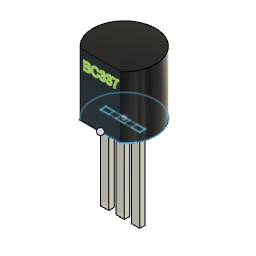
BC337 (Autodesk Fusion 360 design; units mm, degrees)
Autodesk Fusion 360 part; units mm, degrees
sketch "Sketch1" plane through (0, 0, 0) normal (0, 0, 1) x (1, 0, 0)
  line L0 (0, 0) -> (-1.725, 0)
  line L1 (-1.725, 0) -> (-1.725, 0.0215)
  line L2 (1.725, 0) -> (1.725, 0.0215)
  line L3 (0, 0) -> (1.725, 0)
  arc A0 (1.7, 0) -> (-1.7, 0) centre (0, 2) ccw
  line L4 (-1.6, 1.6) -> (1.7, 1.6)
  line L5 (1.7, 1.6) -> (1.7, 2.05)
  line L6 (1.7, 2.05) -> (-1.6, 2.05)
  line L7 (-1.6, 2.05) -> (-1.6, 1.6)
  line L8 (-1.6, 1.6) -> (-0.9, 1.6)
  line L9 (-0.9, 1.6) -> (-0.9, 2.05)
  line L10 (-0.9, 2.05) -> (-1.6, 2.05)
  line L11 (-1.6, 2.05) -> (-1.6, 1.6)
  line L12 (1.7, 2.05) -> (1, 2.05)
  line L13 (1, 2.05) -> (1, 1.6)
  line L14 (1, 1.6) -> (1.7, 1.6)
  line L15 (1.7, 1.6) -> (1.7, 2.05)
  line L16 (-0.2974, 2.05) -> (0.4026, 2.05)
  line L17 (0.4026, 2.05) -> (0.4026, 1.6)
  line L18 (0.4026, 1.6) -> (-0.2974, 1.6)
  line L19 (-0.2974, 1.6) -> (-0.2974, 2.05)
  dimension "d7" = 3.3
  dimension "d8" = 0.45
  dimension "d9" = 0.7
  dimension "d10" = 0.7
  dimension "d11" = 0.7
  constraint coincident L0.start L3.start
  constraint horizontal L0
  constraint perpendicular L0 L1
  constraint coincident L0 A0.end
  constraint coincident L3 A0.start
  constraint coincident A0 L1.end
  constraint coincident A0 L2.end
  constraint horizontal L4
  constraint vertical L5
  constraint horizontal L6
  constraint vertical L7
  constraint horizontal L8
  constraint vertical L9
  constraint horizontal L10
  constraint vertical L11
  constraint horizontal L12
  constraint vertical L13
  constraint horizontal L14
  constraint vertical L15
  constraint horizontal L16
  constraint vertical L17
  constraint horizontal L18
  constraint vertical L19
  constraint coincident L6 L16.start
  measures "d7" distance of L4.start L4.end
  measures "d8" distance of L4.start L6.end
  measures "d9" distance of L4.start L8.end
  measures "d10" distance of L5.end L12.end
  measures "d11" distance of L16.start L16.end
extrude "Extrude2" add sketch "Sketch1" against normal blind 7 contours L4 L5 L6 L12 L13 L14 L15 makes body 1
extrude "Extrude1" add sketch "Sketch1" along normal blind 5.2 separate body contours L0 L3 A0 | L4 L6 L7 L8 L9 L10 L11 | L4 L6 L9 L19 | L4 L6 L16 L17 L18 L19 | L4 L6 L13 L17 | L4 L5 L6 L12 L13 L14 L15 makes body 2
extrude "Extrude3" add sketch "Sketch1" against normal blind 7 contours L4 L6 L16 L17 L18 L19 bodies 2
extrude "Extrude4" add sketch "Sketch1" against normal blind 7 contours L4 L6 L7 L8 L9 L10 L11 bodies 2
sketch "Sketch2" plane through (0, 0, 0) normal (0, -1, 0) x (1, 0, 0)
  line L0 (-1.7, 0) -> (1.7, 0)
  line L1 (1.7, 0) -> (1.7, 5.2)
  line L2 (1.7, 5.2) -> (-1.7, 5.2)
  line L3 (-1.7, 5.2) -> (-1.7, 0)
  line L4 (-1.3801, 3.7908) -> (-1.3801, 4.4908)
  line L5 (-1.3801, 4.4908) -> (-1.1175, 4.4908)
  spline S0 degree 2 poles (-1.1175, 4.4908) (-1.0373, 4.4908) (-0.9888, 4.4696) knots 0 0 0 1 1 1
  spline S1 degree 2 poles (-0.9888, 4.4696) (-0.9403, 4.4483) (-0.9129, 4.4042) knots 0 0 0 1 1 1
  spline S2 degree 2 poles (-0.9129, 4.4042) (-0.8854, 4.36) (-0.8854, 4.3118) knots 0 0 0 1 1 1
  spline S3 degree 2 poles (-0.8854, 4.3118) (-0.8854, 4.2669) (-0.9098, 4.2273) knots 0 0 0 1 1 1
  spline S4 degree 2 poles (-0.9098, 4.2273) (-0.9341, 4.1876) (-0.9833, 4.1633) knots 0 0 0 1 1 1
  spline S5 degree 2 poles (-0.9833, 4.1633) (-0.9198, 4.1447) (-0.8857, 4.0998) knots 0 0 0 1 1 1
  spline S6 degree 2 poles (-0.8857, 4.0998) (-0.8515, 4.0549) (-0.8515, 3.9938) knots 0 0 0 1 1 1
  spline S7 degree 2 poles (-0.8515, 3.9938) (-0.8515, 3.9446) (-0.8723, 3.9023) knots 0 0 0 1 1 1
  spline S8 degree 2 poles (-0.8723, 3.9023) (-0.8931, 3.8601) (-0.9236, 3.8372) knots 0 0 0 1 1 1
  spline S9 degree 2 poles (-0.9236, 3.8372) (-0.9542, 3.8142) (-1.0003, 3.8025) knots 0 0 0 1 1 1
  spline S10 degree 2 poles (-1.0003, 3.8025) (-1.0463, 3.7908) (-1.1132, 3.7908) knots 0 0 0 1 1 1
  line L6 (-1.1132, 3.7908) -> (-1.3801, 3.7908)
  line L7 (-1.2875, 4.1967) -> (-1.1361, 4.1967)
  spline S11 degree 2 poles (-1.1361, 4.1967) (-1.0745, 4.1967) (-1.0478, 4.2048) knots 0 0 0 1 1 1
  spline S12 degree 2 poles (-1.0478, 4.2048) (-1.0124, 4.2153) (-0.9945, 4.2397) knots 0 0 0 1 1 1
  spline S13 degree 2 poles (-0.9945, 4.2397) (-0.9766, 4.264) (-0.9766, 4.3008) knots 0 0 0 1 1 1
  spline S14 degree 2 poles (-0.9766, 4.3008) (-0.9766, 4.3357) (-0.9933, 4.3622) knots 0 0 0 1 1 1
  spline S15 degree 2 poles (-0.9933, 4.3622) (-1.01, 4.3887) (-1.0411, 4.3984) knots 0 0 0 1 1 1
  spline S16 degree 2 poles (-1.0411, 4.3984) (-1.0721, 4.4082) (-1.1476, 4.4082) knots 0 0 0 1 1 1
  line L8 (-1.1476, 4.4082) -> (-1.2875, 4.4082)
  line L9 (-1.2875, 4.4082) -> (-1.2875, 4.1967)
  line L10 (-1.2875, 3.8734) -> (-1.1132, 3.8734)
  spline S17 degree 2 poles (-1.1132, 3.8734) (-1.0683, 3.8734) (-1.0502, 3.8768) knots 0 0 0 1 1 1
  spline S18 degree 2 poles (-1.0502, 3.8768) (-1.0182, 3.8825) (-0.9967, 3.8959) knots 0 0 0 1 1 1
  spline S19 degree 2 poles (-0.9967, 3.8959) (-0.9752, 3.9093) (-0.9613, 3.9348) knots 0 0 0 1 1 1
  spline S20 degree 2 poles (-0.9613, 3.9348) (-0.9475, 3.9603) (-0.9475, 3.9938) knots 0 0 0 1 1 1
  spline S21 degree 2 poles (-0.9475, 3.9938) (-0.9475, 4.0329) (-0.9676, 4.0618) knots 0 0 0 1 1 1
  spline S22 degree 2 poles (-0.9676, 4.0618) (-0.9876, 4.0907) (-1.0232, 4.1024) knots 0 0 0 1 1 1
  spline S23 degree 2 poles (-1.0232, 4.1024) (-1.0588, 4.1141) (-1.1256, 4.1141) knots 0 0 0 1 1 1
  line L11 (-1.1256, 4.1141) -> (-1.2875, 4.1141)
  line L12 (-1.2875, 4.1141) -> (-1.2875, 3.8734)
  line L13 (-0.2246, 4.0363) -> (-0.1319, 4.0129)
  spline S24 degree 2 poles (-0.1319, 4.0129) (-0.1611, 3.8988) (-0.2368, 3.8388) knots 0 0 0 1 1 1
  spline S25 degree 2 poles (-0.2368, 3.8388) (-0.3124, 3.7789) (-0.4218, 3.7789) knots 0 0 0 1 1 1
  spline S26 degree 2 poles (-0.4218, 3.7789) (-0.5349, 3.7789) (-0.6059, 3.825) knots 0 0 0 1 1 1
  spline S27 degree 2 poles (-0.6059, 3.825) (-0.6768, 3.8711) (-0.7138, 3.9584) knots 0 0 0 1 1 1
  spline S28 degree 2 poles (-0.7138, 3.9584) (-0.7508, 4.0458) (-0.7508, 4.1461) knots 0 0 0 1 1 1
  spline S29 degree 2 poles (-0.7508, 4.1461) (-0.7508, 4.2554) (-0.709, 4.3368) knots 0 0 0 1 1 1
  spline S30 degree 2 poles (-0.709, 4.3368) (-0.6672, 4.4183) (-0.5901, 4.4605) knots 0 0 0 1 1 1
  spline S31 degree 2 poles (-0.5901, 4.4605) (-0.513, 4.5028) (-0.4203, 4.5028) knots 0 0 0 1 1 1
  spline S32 degree 2 poles (-0.4203, 4.5028) (-0.3153, 4.5028) (-0.2437, 4.4493) knots 0 0 0 1 1 1
  spline S33 degree 2 poles (-0.2437, 4.4493) (-0.1721, 4.3958) (-0.1439, 4.2989) knots 0 0 0 1 1 1
  line L14 (-0.1439, 4.2989) -> (-0.2351, 4.2774)
  spline S34 degree 2 poles (-0.2351, 4.2774) (-0.2594, 4.3538) (-0.3058, 4.3887) knots 0 0 0 1 1 1
  spline S35 degree 2 poles (-0.3058, 4.3887) (-0.3521, 4.4235) (-0.4223, 4.4235) knots 0 0 0 1 1 1
  spline S36 degree 2 poles (-0.4223, 4.4235) (-0.503, 4.4235) (-0.5571, 4.3848) knots 0 0 0 1 1 1
  spline S37 degree 2 poles (-0.5571, 4.3848) (-0.6113, 4.3462) (-0.6333, 4.281) knots 0 0 0 1 1 1
  spline S38 degree 2 poles (-0.6333, 4.281) (-0.6553, 4.2158) (-0.6553, 4.1466) knots 0 0 0 1 1 1
  spline S39 degree 2 poles (-0.6553, 4.1466) (-0.6553, 4.0573) (-0.6292, 3.9907) knots 0 0 0 1 1 1
  spline S40 degree 2 poles (-0.6292, 3.9907) (-0.6032, 3.9241) (-0.5483, 3.8911) knots 0 0 0 1 1 1
  spline S41 degree 2 poles (-0.5483, 3.8911) (-0.4934, 3.8582) (-0.4294, 3.8582) knots 0 0 0 1 1 1
  spline S42 degree 2 poles (-0.4294, 3.8582) (-0.3516, 3.8582) (-0.2976, 3.903) knots 0 0 0 1 1 1
  spline S43 degree 2 poles (-0.2976, 3.903) (-0.2437, 3.9479) (-0.2246, 4.0363) knots 0 0 0 1 1 1
  line L15 (-0.0522, 3.9756) -> (0.0337, 3.9871)
  spline S44 degree 2 poles (0.0337, 3.9871) (0.0485, 3.914) (0.0841, 3.8818) knots 0 0 0 1 1 1
  spline S45 degree 2 poles (0.0841, 3.8818) (0.1197, 3.8496) (0.1708, 3.8496) knots 0 0 0 1 1 1
  spline S46 degree 2 poles (0.1708, 3.8496) (0.2314, 3.8496) (0.2732, 3.8916) knots 0 0 0 1 1 1
  spline S47 degree 2 poles (0.2732, 3.8916) (0.315, 3.9336) (0.315, 3.9957) knots 0 0 0 1 1 1
  spline S48 degree 2 poles (0.315, 3.9957) (0.315, 4.0549) (0.2763, 4.0933) knots 0 0 0 1 1 1
  spline S49 degree 2 poles (0.2763, 4.0933) (0.2376, 4.1318) (0.1779, 4.1318) knots 0 0 0 1 1 1
  spline S50 degree 2 poles (0.1779, 4.1318) (0.1536, 4.1318) (0.1173, 4.1222) knots 0 0 0 1 1 1
  line L16 (0.1173, 4.1222) -> (0.1269, 4.1977)
  spline S51 degree 2 poles (0.1269, 4.1977) (0.1355, 4.1967) (0.1407, 4.1967) knots 0 0 0 1 1 1
  spline S52 degree 2 poles (0.1407, 4.1967) (0.1956, 4.1967) (0.2395, 4.2254) knots 0 0 0 1 1 1
  spline S53 degree 2 poles (0.2395, 4.2254) (0.2835, 4.254) (0.2835, 4.3137) knots 0 0 0 1 1 1
  spline S54 degree 2 poles (0.2835, 4.3137) (0.2835, 4.361) (0.2515, 4.392) knots 0 0 0 1 1 1
  spline S55 degree 2 poles (0.2515, 4.392) (0.2195, 4.423) (0.1689, 4.423) knots 0 0 0 1 1 1
  spline S56 degree 2 poles (0.1689, 4.423) (0.1187, 4.423) (0.0853, 4.3915) knots 0 0 0 1 1 1
  spline S57 degree 2 poles (0.0853, 4.3915) (0.0519, 4.36) (0.0423, 4.297) knots 0 0 0 1 1 1
  line L17 (0.0423, 4.297) -> (-0.0436, 4.3123)
  spline S58 degree 2 poles (-0.0436, 4.3123) (-0.0279, 4.3987) (0.028, 4.4462) knots 0 0 0 1 1 1
  spline S59 degree 2 poles (0.028, 4.4462) (0.0839, 4.4937) (0.167, 4.4937) knots 0 0 0 1 1 1
  spline S60 degree 2 poles (0.167, 4.4937) (0.2243, 4.4937) (0.2725, 4.4691) knots 0 0 0 1 1 1
  spline S61 degree 2 poles (0.2725, 4.4691) (0.3207, 4.4445) (0.3463, 4.402) knots 0 0 0 1 1 1
  spline S62 degree 2 poles (0.3463, 4.402) (0.3718, 4.3595) (0.3718, 4.3118) knots 0 0 0 1 1 1
  spline S63 degree 2 poles (0.3718, 4.3118) (0.3718, 4.2664) (0.3475, 4.2292) knots 0 0 0 1 1 1
  spline S64 degree 2 poles (0.3475, 4.2292) (0.3231, 4.1919) (0.2754, 4.17) knots 0 0 0 1 1 1
  spline S65 degree 2 poles (0.2754, 4.17) (0.3374, 4.1556) (0.3718, 4.1105) knots 0 0 0 1 1 1
  spline S66 degree 2 poles (0.3718, 4.1105) (0.4062, 4.0654) (0.4062, 3.9976) knots 0 0 0 1 1 1
  spline S67 degree 2 poles (0.4062, 3.9976) (0.4062, 3.9059) (0.3393, 3.8422) knots 0 0 0 1 1 1
  spline S68 degree 2 poles (0.3393, 3.8422) (0.2725, 3.7784) (0.1703, 3.7784) knots 0 0 0 1 1 1
  spline S69 degree 2 poles (0.1703, 3.7784) (0.0782, 3.7784) (0.0173, 3.8333) knots 0 0 0 1 1 1
  spline S70 degree 2 poles (0.0173, 3.8333) (-0.0436, 3.8882) (-0.0522, 3.9756) knots 0 0 0 1 1 1
  line L18 (0.4917, 3.9756) -> (0.5776, 3.9871)
  spline S71 degree 2 poles (0.5776, 3.9871) (0.5924, 3.914) (0.628, 3.8818) knots 0 0 0 1 1 1
  spline S72 degree 2 poles (0.628, 3.8818) (0.6636, 3.8496) (0.7146, 3.8496) knots 0 0 0 1 1 1
  spline S73 degree 2 poles (0.7146, 3.8496) (0.7753, 3.8496) (0.8171, 3.8916) knots 0 0 0 1 1 1
  spline S74 degree 2 poles (0.8171, 3.8916) (0.8588, 3.9336) (0.8588, 3.9957) knots 0 0 0 1 1 1
  spline S75 degree 2 poles (0.8588, 3.9957) (0.8588, 4.0549) (0.8202, 4.0933) knots 0 0 0 1 1 1
  spline S76 degree 2 poles (0.8202, 4.0933) (0.7815, 4.1318) (0.7218, 4.1318) knots 0 0 0 1 1 1
  spline S77 degree 2 poles (0.7218, 4.1318) (0.6975, 4.1318) (0.6612, 4.1222) knots 0 0 0 1 1 1
  line L19 (0.6612, 4.1222) -> (0.6707, 4.1977)
  spline S78 degree 2 poles (0.6707, 4.1977) (0.6793, 4.1967) (0.6846, 4.1967) knots 0 0 0 1 1 1
  spline S79 degree 2 poles (0.6846, 4.1967) (0.7395, 4.1967) (0.7834, 4.2254) knots 0 0 0 1 1 1
  spline S80 degree 2 poles (0.7834, 4.2254) (0.8273, 4.254) (0.8273, 4.3137) knots 0 0 0 1 1 1
  spline S81 degree 2 poles (0.8273, 4.3137) (0.8273, 4.361) (0.7953, 4.392) knots 0 0 0 1 1 1
  spline S82 degree 2 poles (0.7953, 4.392) (0.7633, 4.423) (0.7127, 4.423) knots 0 0 0 1 1 1
  spline S83 degree 2 poles (0.7127, 4.423) (0.6626, 4.423) (0.6292, 4.3915) knots 0 0 0 1 1 1
  spline S84 degree 2 poles (0.6292, 4.3915) (0.5958, 4.36) (0.5862, 4.297) knots 0 0 0 1 1 1
  line L20 (0.5862, 4.297) -> (0.5003, 4.3123)
  spline S85 degree 2 poles (0.5003, 4.3123) (0.516, 4.3987) (0.5719, 4.4462) knots 0 0 0 1 1 1
  spline S86 degree 2 poles (0.5719, 4.4462) (0.6277, 4.4937) (0.7108, 4.4937) knots 0 0 0 1 1 1
  spline S87 degree 2 poles (0.7108, 4.4937) (0.7681, 4.4937) (0.8164, 4.4691) knots 0 0 0 1 1 1
  spline S88 degree 2 poles (0.8164, 4.4691) (0.8646, 4.4445) (0.8901, 4.402) knots 0 0 0 1 1 1
  spline S89 degree 2 poles (0.8901, 4.402) (0.9157, 4.3595) (0.9157, 4.3118) knots 0 0 0 1 1 1
  spline S90 degree 2 poles (0.9157, 4.3118) (0.9157, 4.2664) (0.8913, 4.2292) knots 0 0 0 1 1 1
  spline S91 degree 2 poles (0.8913, 4.2292) (0.867, 4.1919) (0.8192, 4.17) knots 0 0 0 1 1 1
  spline S92 degree 2 poles (0.8192, 4.17) (0.8813, 4.1556) (0.9157, 4.1105) knots 0 0 0 1 1 1
  spline S93 degree 2 poles (0.9157, 4.1105) (0.95, 4.0654) (0.95, 3.9976) knots 0 0 0 1 1 1
  spline S94 degree 2 poles (0.95, 3.9976) (0.95, 3.9059) (0.8832, 3.8422) knots 0 0 0 1 1 1
  spline S95 degree 2 poles (0.8832, 3.8422) (0.8164, 3.7784) (0.7142, 3.7784) knots 0 0 0 1 1 1
  spline S96 degree 2 poles (0.7142, 3.7784) (0.622, 3.7784) (0.5611, 3.8333) knots 0 0 0 1 1 1
  spline S97 degree 2 poles (0.5611, 3.8333) (0.5003, 3.8882) (0.4917, 3.9756) knots 0 0 0 1 1 1
  line L21 (1.0408, 4.3992) -> (1.0408, 4.4818)
  line L22 (1.0408, 4.4818) -> (1.4939, 4.4818)
  line L23 (1.4939, 4.4818) -> (1.4939, 4.4149)
  spline S98 degree 2 poles (1.4939, 4.4149) (1.4271, 4.3438) (1.3614, 4.2258) knots 0 0 0 1 1 1
  spline S99 degree 2 poles (1.3614, 4.2258) (1.2958, 4.1079) (1.2599, 3.9833) knots 0 0 0 1 1 1
  spline S100 degree 2 poles (1.2599, 3.9833) (1.2342, 3.8954) (1.227, 3.7908) knots 0 0 0 1 1 1
  line L24 (1.227, 3.7908) -> (1.1387, 3.7908)
  spline S101 degree 2 poles (1.1387, 3.7908) (1.1401, 3.8734) (1.1711, 3.9904) knots 0 0 0 1 1 1
  spline S102 degree 2 poles (1.1711, 3.9904) (1.2022, 4.1074) (1.2602, 4.216) knots 0 0 0 1 1 1
  spline S103 degree 2 poles (1.2602, 4.216) (1.3182, 4.3247) (1.3836, 4.3992) knots 0 0 0 1 1 1
  line L25 (1.3836, 4.3992) -> (1.0408, 4.3992)
